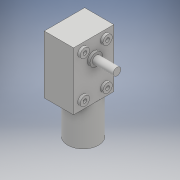
# Autodesk Inventor part: Мотор
Saved by Autodesk Inventor 2017 (Build 210142000, 142)
## iProperties
Part Number: Мотор
Material: Типовые
Document SubType Name: Modeling
Designer: Daemon
Density: 1 g/cm^3
Appearance: По умолчанию
Author: Daemon
Autodesk Inventor part; units mm, degrees
ref_plane "XZ Plane" through (0, 0, 0) normal (0, 1, 0) x (-1, 0, 0)
sketch "Эскиз1" plane through (0, 0, 0) normal (0, 0, 1) x (1, 0, 0)
  circle A0 centre (0, 0) radius 12.2
  dimension "d0" = 24.4
  constraints: 1 centre point, 1 coincident
  measures "d0" diameter of A0
extrude "Выдавливание1" add sketch "Эскиз1" along normal blind 30.8
ref_plane "РабПлоскость1" through (12.2, 0, 0) normal (1, 0, 0) x (0, 1, 0)
sketch "Эскиз2" plane through (12.2, 0, 0) normal (1, 0, 0) x (0, 1, 0)
  line L0 (12.2, 0) -> (12.2, 30.8) projected
  line L1 (12.2, 30.8) -> (-19.8, 30.8)
  line L2 (-19.8, 30.8) -> (-19.8, 76.8)
  line L3 (-19.8, 76.8) -> (12.2, 76.8)
  line L4 (12.2, 76.8) -> (12.2, 30.8)
  point P0 (0, 0)
  dimension "d3" = 46
  dimension "d4" = 32
  constraints: 8 end point, 2 parallel, 1 horizontal, 1 perpendicular, 1 point on line
  measures "d3" distance of L3.end L1.start
  measures "d4" distance of L2.end L3.end
extrude "Выдавливание2" add sketch "Эскиз2" against normal blind 23.2
sketch "Эскиз3" plane through (12.2, 0, 0) normal (1, 0, 0) x (0, 0, -1)
  circle A0 centre (-70.8, -12.8) radius 3.7
  line L0 (0, 0) -> (0, -12.8)
  line L1 (0, -12.8) -> (-70.8, -12.8)
  point P0 (-76.8, -19.8)
  dimension "d10" = 7.4
  dimension "d11" = 12.8
  dimension "d12" = 70.8
  constraints: 4 end point, 1 centre point, 1 perpendicular, 1 vertical
  measures "d10" diameter of A0
  measures "d11" distance from line of L0.start L1
  measures "d12" distance from line of L1.end L0
extrude "Выдавливание3" add sketch "Эскиз3" along normal blind 2
ref_plane "РабПлоскость2" through (12.2, -3.8, 30.8) normal (0, -1, 0) x (1, 0, 0)
mirror "Зеркальное отражение1" about plane through (12.2, -3.8, 30.8) normal (0, -1, 0) of "Выдавливание3"
sketch "Эскиз4" plane through (12.2, 0, 0) normal (1, 0, 0) x (0, 0, -1)
  line L0 (-30.8, -5.2764) -> (-30.8, -19.8) projected
  line L1 (-30.8, -19.8) -> (-37.8, -19.8)
  line L2 (-30.8, -19.8) -> (-76.8, -19.8) projected
  line L3 (-37.8, -19.8) -> (-37.8, -12.8)
  circle A0 centre (-37.8, -12.8) radius 3.7
  point P0 (0, 0)
  dimension "d15" = 7
  dimension "d16" = 7
  dimension "d17" = 7.4
  constraints: 4 end point, 1 centre point, 1 coincident, 1 point on line, 1 vertical
  measures "d15" distance of L0.end L1.end
  measures "d16" distance of L1.end L3.end
  measures "d17" diameter of A0
extrude "Выдавливание4" add sketch "Эскиз4" along normal blind 2
mirror "Зеркальное отражение2" about plane through (12.2, -3.8, 30.8) normal (0, -1, 0) of "Выдавливание4"
sketch "Эскиз5" plane through (12.2, 0, 0) normal (1, 0, 0) x (0, 0, -1)
  circle A0 centre (-70.8, -12.8) radius 3.7 projected
  circle A1 centre (-70.8, 5.2) radius 3.7 projected
  line L0 (-76.8, -19.8) -> (-61.8, -19.8)
  line L1 (-61.8, -19.8) -> (-61.8, -3.8)
  circle A2 centre (-61.8, -3.8) radius 3
  point P0 (0, 0)
  dimension "d20" = 15
  dimension "d21" = 16
  dimension "d22" = 6
  constraints: 4 end point, 1 centre point, 1 coincident, 1 vertical
  measures "d20" distance of L0.start L0.end
  measures "d21" distance of L0.end L1.end
  measures "d22" diameter of A2
extrude "Выдавливание5" add sketch "Эскиз5" along normal blind 18.5 contours A2
sketch "Эскиз6" plane through (14.2, -12.8, 70.8) normal (1, 0, 0) x (0, 0, -1)
  circle A0 centre (0, 0) radius 3.7 projected
  circle A1 centre (0, 0) radius 1.5
  point P0 (70.8, 12.8)
  dimension "d25" = 3
  constraints: 1 centre point, 1 coincident
  measures "d25" diameter of A1
extrude "Выдавливание6" cut sketch "Эскиз6" against normal blind 2 contours A1
mirror "Зеркальное отражение3" about plane through (12.2, -3.8, 30.8) normal (0, -1, 0) of "Выдавливание6"
sketch "Эскиз8" plane through (14.2, -12.8, 37.8) normal (1, 0, 0) x (0, 0, -1)
  circle A0 centre (0, 0) radius 3.7 projected
  circle A1 centre (0, 0) radius 1.5
  point P0 (37.8, 12.8)
  dimension "d28" = 3
  constraints: 1 centre point, 1 coincident
  measures "d28" diameter of A1
extrude "Выдавливание7" cut sketch "Эскиз8" against normal blind 2 contours A1
mirror "Зеркальное отражение4" about plane through (12.2, -3.8, 30.8) normal (0, -1, 0) of "Выдавливание7"
sketch "Эскиз9" plane through (12.2, 0, 0) normal (1, 0, 0) x (0, 0, -1)
  circle A0 centre (-61.8, -3.8) radius 3 projected
  circle A1 centre (-61.8, -3.8) radius 5
  point P0 (0, 0)
  dimension "d31" = 10
  constraints: 1 centre point, 1 coincident
  measures "d31" diameter of A1
extrude "Выдавливание8" add sketch "Эскиз9" along normal blind 2
